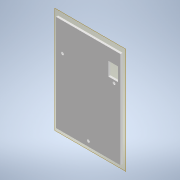
# Autodesk Inventor part: top
Saved by Autodesk Inventor 2022 (Build 260153000, 153)
## iProperties
Created: 2022-10-20
Part Number: top
Material: Типовые
Document SubType Name: Modeling
Designer: Robo0
Density: 1 g/cm^3
Appearance: По умолчанию
Author: Robo0
Autodesk Inventor part; units mm, degrees
ref_plane "YZ Plane" through (0, 0, 0) normal (1, 0, 0) x (0, 1, 0)
ref_plane "XZ Plane" through (0, 0, 0) normal (0, 1, 0) x (-1, 0, 0)
ref_plane "XY Plane" through (0, 0, 0) normal (0, 0, 1) x (1, 0, 0)
ref_plane "РабПлоскость1" through (0, 0, 0) normal (0, 0, 1) x (1, 0, 0)
sketch "Эскиз1" plane through (0, 0, 0) normal (0, 0, 1) x (1, 0, 0)
  line L0 (45.389, -67.917) -> (45.389, 67.917)
  line L1 (45.389, 67.917) -> (-45.389, 67.917)
  line L2 (-45.389, -67.917) -> (45.389, -67.917)
  line L3 (-45.389, 67.917) -> (-45.389, -67.917)
  line L4 (41.8047, 51.1354) -> (28.1516, 51.1354)
  line L5 (28.1516, 51.1354) -> (28.1516, 31.897)
  line L6 (28.1516, 31.897) -> (41.8047, 31.897)
  line L7 (41.8047, 31.897) -> (41.8047, 51.1354)
  circle A0 centre (36.389, 27.7057) radius 2.75
  circle A1 centre (0, -60.917) radius 2.75
  circle A2 centre (-36.389, 27.7057) radius 2.75
  circle A3 centre (36.389, 27.7057) radius 2
  circle A4 centre (0, -60.917) radius 2
  circle A5 centre (-36.389, 27.7057) radius 2
  point P0 (0, 0)
extrude "Выдавливание1" add sketch "Эскиз1" along normal blind 3 contours L2 L3 L1 L0 | A0 | A1 | A2
sketch "Эскиз2" plane through (0, 0, 0) normal (0, 0, -1) x (-1, 0, 0)
  line L0 (42.389, -64.917) -> (-42.389, -64.917) projected
  line L1 (-42.389, -64.917) -> (-42.389, 54.5577) projected
  line L2 (-42.611, 64.083) -> (10.389, 64.083) projected
  line L3 (42.389, 64.917) -> (42.389, -64.917) projected
  line L4 (-32.389, -64.917) -> (-12.389, -64.917)
  line L5 (-12.389, -64.917) -> (-12.389, -62.917)
  line L6 (-12.389, -62.917) -> (-32.389, -62.917)
  line L7 (-32.389, -62.917) -> (-32.389, -64.917)
  line L8 (-32.389, 64.083) -> (-12.389, 64.083)
  line L9 (-12.389, 64.083) -> (-12.389, 62.083)
  line L10 (-12.389, 62.083) -> (-32.389, 62.083)
  line L11 (-32.389, 62.083) -> (-32.389, 64.083)
  line L12 (-32.389, 62.083) -> (-12.389, 62.083)
  line L13 (-12.389, 62.083) -> (-12.389, 60.083)
  line L14 (-12.389, 60.083) -> (-32.389, 60.083)
  line L15 (-32.389, 60.083) -> (-32.389, 62.083)
  line L16 (42.389, -10) -> (40.389, -10)
  line L17 (40.389, -10) -> (40.389, 10)
  line L18 (40.389, 10) -> (42.389, 10)
  line L19 (42.389, 10) -> (42.389, -10)
  point P0 (0, 0)
  point P1 (-12.389, 64.083)
  dimension "d5" = 20
  dimension "d6" = 10
  dimension "d7" = 2
  dimension "d8" = 2
  dimension "d9" = 2
  dimension "d10" = 2
  dimension "d11" = 20
  dimension "d12" = 10
  constraints: 32 end point, 8 parallel, 5 point on line, 4 horizontal, 4 perpendicular
  measures "d5" distance of L5.end L6.end
  measures "d6" distance from line of L6.end L1
  measures "d7" distance between parallel lines of L0 L6
  measures "d8" distance between parallel lines of L14 L10
  measures "d9" distance between parallel lines of L10 L2
  measures "d10" distance between parallel lines of L19 L17
  measures "d11" distance from line of L16.end L18
  measures "d12" vertical distance of point (0, 0) L17.end
extrude "Выдавливание2" add sketch "Эскиз2" along normal blind 2 contours L0 L7 L6 L5 | L2 L9 L10 L11 | L3 L16 L17 L18
equation "\"d9\" = d8"
